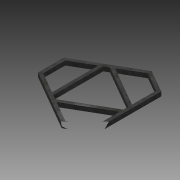
# Autodesk Inventor part: BasePlatform
Saved by Autodesk Inventor 2015 SP1 (Build 190203100, 203)
## iProperties
Created: 2016-02-02
Part Number: BasePlatform
Material: Steel
Document SubType Name: Modeling
Designer: tuttlem
Mass: 32237.8 g
Surface Area: 4761.07 cm^2
Volume: 4106.72 cm^3
Density: 7.85 g/cm^3
Appearance: Plate
Author: tuttlem
Autodesk Inventor part; units mm, degrees
ref_plane "YZ Plane" through (0, 0, 0) normal (1, 0, 0) x (0, 1, 0)
ref_plane "XZ Plane" through (0, 0, 0) normal (0, 1, 0) x (-1, 0, 0)
ref_plane "XY Plane" through (0, 0, 0) normal (0, 0, 1) x (1, 0, 0)
sketch "Sketch1" plane through (0, 0, 0) normal (0, 1, 0) x (-1, 0, 0)
  line L0 (908.9386, 54.09) -> (249.0272, 435.09)
  line L1 (-14.9373, 282.69) -> (-14.9373, -479.31)
  line L2 (249.0272, -631.71) -> (908.9386, -250.71)
  line L3 (908.9386, 54.09) -> (908.9386, -250.71)
  line L4 (249.0272, 435.09) -> (-14.9373, 282.69)
  line L5 (249.0272, -631.71) -> (-14.9373, -479.31)
  line L6 (870.8386, 32.0929) -> (249.0272, 391.0959)
  line L7 (249.0272, 391.0959) -> (23.1627, 260.6929)
  line L8 (23.1627, 260.6929) -> (23.1627, -457.313)
  line L9 (23.1627, -457.313) -> (249.0272, -587.7159)
  line L10 (249.0272, -587.7159) -> (870.8386, -228.713)
  line L11 (870.8386, -228.713) -> (870.8386, 32.0929)
  line L12 (585.2718, 196.965) -> (585.2718, -393.585)
  line L13 (534.594, 226.2238) -> (23.1627, -69.0512)
  line L14 (534.594, -422.8439) -> (23.1627, -127.5689)
  line L15 (496.494, 248.2209) -> (23.1627, -25.0571)
  line L16 (23.1627, -171.563) -> (496.494, -444.8409)
  line L17 (623.3718, 174.9679) -> (623.3718, -371.588)
  line L18 (-156.6121, -547.5732) -> (-156.6121, 528.0779)
  line L19 (-1222.1628, 54.09) -> (-562.2514, 435.09)
  line L20 (-298.2869, 282.69) -> (-298.2869, -479.31)
  line L21 (-562.2514, -631.71) -> (-1222.1628, -250.71)
  line L22 (-1222.1628, 54.09) -> (-1222.1628, -250.71)
  line L23 (-562.2514, 435.09) -> (-298.2869, 282.69)
  line L24 (-562.2514, -631.71) -> (-298.2869, -479.31)
  line L25 (-1184.0628, 32.0929) -> (-562.2514, 391.0959)
  line L26 (-562.2514, 391.0959) -> (-336.3869, 260.6929)
  line L27 (-336.3869, 260.6929) -> (-336.3869, -457.313)
  line L28 (-336.3869, -457.313) -> (-562.2514, -587.7159)
  line L29 (-562.2514, -587.7159) -> (-1184.0628, -228.713)
  line L30 (-1184.0628, -228.713) -> (-1184.0628, 32.0929)
  line L31 (-898.496, 196.965) -> (-898.496, -393.585)
  line L32 (-847.8182, 226.2238) -> (-336.3869, -69.0512)
  line L33 (-847.8182, -422.8439) -> (-336.3869, -127.5689)
  line L34 (-809.7182, 248.2209) -> (-336.3869, -25.0571)
  line L35 (-336.3869, -171.563) -> (-809.7182, -444.8409)
  line L36 (-936.596, 174.9679) -> (-936.596, -371.588)
  constraints: 74 end point, 24 point on line, 24 symmetric about line, 16 parallel
extrude "Extrusion1" add sketch "Sketch1" along normal blind 50.8 contours L3 L2 L5 L1 L4 L0 | L17 L10 L12 L6 | L13 L8 L15 L6 | L10 L16 L8 L14
body "Solid1"
